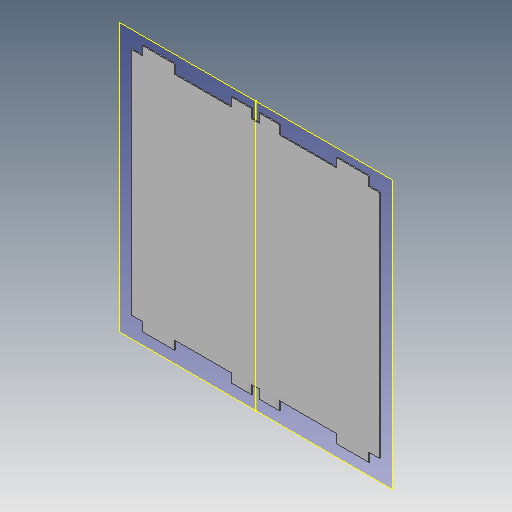
# Autodesk Inventor part: mid_heater
Saved by Autodesk Inventor 2020 (Build 240168000, 168)
## iProperties
Created: 2021-05-08
Part Number: mid_heater
Material: Generic
Document SubType Name: Modeling
Designer: Hsu Daniel
Density: 1 g/cm^3
Appearance: Default
Author: Hsu Daniel
Autodesk Inventor part; units mm, degrees
ref_plane "YZ Plane" through (0, 0, 0) normal (1, 0, 0) x (0, 1, 0)
ref_plane "XZ Plane" through (0, 0, 0) normal (0, 1, 0) x (-1, 0, 0)
ref_plane "XY Plane" through (0, 0, 0) normal (0, 0, 1) x (1, 0, 0)
sketch "Sketch1" plane through (0, 0, 0) normal (0, 0, 1) x (1, 0, 0)
  line L0 (0, 0) -> (126.6, 0)
  line L1 (63.3, 0) -> (63.3, 10.109) construction
  line L2 (5.5, 0) -> (5.5, -4.5)
  line L3 (5.5, -4.5) -> (22.1, -4.5)
  line L4 (22.1, -4.5) -> (22.1, 0)
  line L5 (50.95, 0) -> (50.95, -4.5)
  line L6 (50.95, -4.5) -> (75.65, -4.5)
  line L7 (75.65, -4.5) -> (75.65, 0)
  line L8 (104.5, 0) -> (104.5, -4.5)
  line L9 (104.5, -4.5) -> (121.1, -4.5)
  line L10 (121.1, -4.5) -> (121.1, 0)
  line L11 (13.8, -4.5) -> (13.8, 0) construction
  line L12 (63.3, -4.5) -> (63.3, 0) construction
  line L13 (112.8, -4.5) -> (112.8, 0) construction
  line L14 (0, 0) -> (0, 58.65)
  line L15 (0, 58.65) -> (126.6, 58.65) construction
  line L16 (126.6, 0) -> (126.6, 58.65)
  line L17 (0, 117.3) -> (126.6, 117.3)
  line L18 (63.3, 117.3) -> (63.3, 107.191) construction
  line L19 (5.5, 117.3) -> (5.5, 121.8)
  line L20 (5.5, 121.8) -> (22.1, 121.8)
  line L21 (22.1, 121.8) -> (22.1, 117.3)
  line L22 (50.95, 117.3) -> (50.95, 121.8)
  line L23 (50.95, 121.8) -> (75.65, 121.8)
  line L24 (75.65, 121.8) -> (75.65, 117.3)
  line L25 (104.5, 117.3) -> (104.5, 121.8)
  line L26 (104.5, 121.8) -> (121.1, 121.8)
  line L27 (121.1, 121.8) -> (121.1, 117.3)
  line L28 (13.8, 121.8) -> (13.8, 117.3) construction
  line L29 (63.3, 121.8) -> (63.3, 117.3) construction
  line L30 (112.8, 121.8) -> (112.8, 117.3) construction
  line L31 (0, 117.3) -> (0, 58.65)
  line L32 (126.6, 117.3) -> (126.6, 58.65)
  dimension "d0" = 126.6
  dimension "d1" = 4.5
  dimension "d2" = 16.6
  dimension "d3" = 4.5
  dimension "d4" = 24.7
  dimension "d5" = 4.5
  dimension "d6" = 16.6
  dimension "d7" = 49.5
  dimension "d8" = 49.5
  dimension "d9" = 58.65
  constraints: 62 end point, 22 symmetric about line, 9 vertical, 8 point on line, 3 midpoint, 2 perpendicular, 1 collinear, 1 horizontal, 25 other
  measures "d0" distance of L14.start L16.start
  measures "d1" distance of L2.start L2.end
  measures "d2" distance of L2.end L3.end
  measures "d3" distance of L5.start L5.end
  measures "d4" distance of L5.end L6.end
  measures "d5" distance of L8.start L8.end
  measures "d6" distance of L8.end L9.end
  measures "d7" distance from line of L11 L12.end
  measures "d8" distance between parallel lines of L13 L12
  measures "d9" distance of L14.start L14.end
extrude "Extrusion1" add sketch "Sketch1" along normal blind 0.5
ref_plane "Work Plane1" through (0, 0, 0.25) normal (0, 0, -1) x (-1, 0, 0)
ref_plane "Work Plane2" through (63.3, 0, 0) normal (1, 0, 0) x (0, 0, -1)
sketch "Sketch2" plane through (0, 0, 0.5) normal (0, 0, 1) x (1, 0, 0)
  line L0 (5.5, 117.3) -> (0, 117.3) projected
  line L1 (0, 117.3) -> (0, 0) projected
  line L2 (0, 0) -> (5.5, 0) projected
  line L3 (5.5, 0) -> (5.5, -4.5) projected
  line L4 (5.5, -4.5) -> (22.1, -4.5) projected
  line L5 (22.1, -4.5) -> (22.1, 0) projected
  line L6 (22.1, 0) -> (50.95, 0) projected
  line L7 (50.95, 0) -> (50.95, -4.5) projected
  line L8 (50.95, -4.5) -> (75.65, -4.5) projected
  line L9 (75.65, -4.5) -> (75.65, 0) projected
  line L10 (75.65, 0) -> (104.5, 0) projected
  line L11 (104.5, 0) -> (104.5, -4.5) projected
  line L12 (104.5, -4.5) -> (121.1, -4.5) projected
  line L13 (121.1, -4.5) -> (121.1, 0) projected
  line L14 (121.1, 0) -> (126.6, 0) projected
  line L15 (126.6, 0) -> (126.6, 117.3) projected
  line L16 (126.6, 117.3) -> (121.1, 117.3) projected
  line L17 (121.1, 117.3) -> (121.1, 121.8) projected
  line L18 (121.1, 121.8) -> (104.5, 121.8) projected
  line L19 (104.5, 121.8) -> (104.5, 117.3) projected
  line L20 (104.5, 117.3) -> (75.65, 117.3) projected
  line L21 (75.65, 117.3) -> (75.65, 121.8) projected
  line L22 (75.65, 121.8) -> (50.95, 121.8) projected
  line L23 (50.95, 121.8) -> (50.95, 117.3) projected
  line L24 (50.95, 117.3) -> (22.1, 117.3) projected
  line L25 (22.1, 117.3) -> (22.1, 121.8) projected
  line L26 (22.1, 121.8) -> (5.5, 121.8) projected
  line L27 (5.5, 121.8) -> (5.5, 117.3) projected
  line L28 (50.95, -4.5) -> (75.65, -4.5) construction
  line L29 (50.95, -4.5) -> (75.65, -4.5) construction
  line L30 (61.4, -4.5) -> (61.4, 0)
  line L31 (61.4, 117.3) -> (61.4, 121.8)
  line L32 (63.3, -4.5) -> (63.3, 0)
  line L33 (63.3, 117.3) -> (63.3, 121.8)
  line L34 (65.2, -4.5) -> (65.2, 0)
  line L35 (65.2, 117.3) -> (65.2, 121.8)
  line L36 (61.4, 117.3) -> (65.2, 117.3)
  line L37 (61.4, 0) -> (65.2, 0)
  constraints: 16 end point, 8 parallel, 6 point on line, 2 horizontal, 2 midpoint
extrude "Extrusion2" cut sketch "Sketch2" against normal blind 0.5 contours L22 L33 L36 L31 | L22 L35 L36 L33 | L30 L37 L32 L8 | L32 L37 L34 L8
equation "\"d0\" = mltotal"
equation "\"d1\" = mdepth"
equation "\"d2\" = mlr"
equation "\"d3\" = mdepth"
equation "\"d4\" = mmid"
equation "\"d5\" = mdepth"
equation "\"d6\" = mlr"
equation "\"d8\" = d7"
equation "\"d9\" = 0.5 * heaterH"
equation "\"d10\" = thick"
equation "\"thick\" = 0.5"
equation "\"lrlr\" = 19"
equation "\"lrmid\" = 19.9"
equation "\"lrdepth\" = 3.3"
equation "\"mlr\" = 16.6"
equation "\"mmid\" = 24.7"
equation "\"mdepth\" = 4.5"
equation "\"lrltotal\" = 126.6"
equation "\"mltotal\" = 126.6"
equation "\"lrbetween\" = 52.1"
equation "\"mbetween\" = 49.5"
equation "\"toler\" = 1"
equation "\"stuckw\" = 6"
equation "\"tight\" = 0.08"
equation "\"sidewallL\" = 132.6"
equation "\"heaterH\" = 117.3"
equation "\"stickL\" = 3.5"
equation "\"wireH\" = 25"
body "Solid1"
